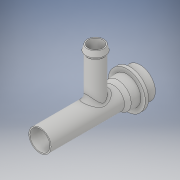
# Autodesk Inventor part: CheckBallonWindbox Connecter 1.0
Saved by Autodesk Inventor 2019 (Build 230136000, 136)
## iProperties
Created: 2019-04-04
Part Number: CheckBallonWindbox Connecter 1.0
Material: Generic
Document SubType Name: Modeling
Designer: Kepler
Density: 1 g/cm^3
Appearance: Default
Author: Kepler
Autodesk Inventor part; units mm, degrees
ref_plane "YZ Plane" through (0, 0, 0) normal (1, 0, 0) x (0, 1, 0)
ref_plane "XZ Plane" through (0, 0, 0) normal (0, 1, 0) x (-1, 0, 0)
ref_plane "XY Plane" through (0, 0, 0) normal (0, 0, 1) x (1, 0, 0)
sketch "Sketch1" plane through (0, 0, 0) normal (0, 0, 1) x (1, 0, 0)
  circle A0 centre (0, 0) radius 10
  circle A1 centre (0, 0) radius 9
  dimension "d0" = 20
  dimension "d1" = 18
  constraints: 3 coincident, 2 centre point
  measures "d0" diameter of A0
  measures "d1" diameter of A1
extrude "Extrusion1" add sketch "Sketch1" along normal blind 50
sketch "Sketch2" plane through (0, 0, 0) normal (0, 0, -1) x (-1, 0, 0)
  circle A0 centre (0, 0) radius 10
  circle A1 centre (0, 0) radius 9
  dimension "d4" = 20
  dimension "d5" = 18
  constraints: 2 centre point, 2 coincident
  measures "d4" diameter of A0
  measures "d5" diameter of A1
extrude "Extrusion2" add sketch "Sketch2" along normal blind 20
sketch "Sketch3" plane through (0, 0, 0) normal (0, 1, 0) x (-1, 0, 0)
  circle A0 centre (0, 0) radius 7.5
  circle A1 centre (0, 0) radius 6.5
  dimension "d8" = 15
  dimension "d9" = 13
  constraints: 2 centre point, 2 coincident
  measures "d8" diameter of A0
  measures "d9" diameter of A1
extrude "Extrusion3" add sketch "Sketch3" along normal blind 50
sketch "Sketch4" plane through (0, 0, 0) normal (0, -1, 0) x (1, 0, 0)
  circle A0 centre (0, 0) radius 6.5
  dimension "d12" = 13
  constraints: 1 centre point, 1 coincident
  measures "d12" diameter of A0
extrude "Extrusion4" cut sketch "Sketch4" against normal blind 20
sketch "Sketch5" plane through (0, 0, -20) normal (0, 0, -1) x (-1, 0, 0)
  circle A0 centre (0, 0) radius 9
  dimension "d15" = 18
  constraints: 1 centre point, 1 coincident
  measures "d15" diameter of A0
extrude "Extrusion5" cut sketch "Sketch5" against normal blind 30
fillet "Fillet1" radius 2 2 edges at (-0.0257, 9, 6.4999) (0.0257, 9, -6.4999)
fillet "Fillet2" radius 4 2 edges at (0.0316, 10, -7.4999) (-0.0297, 10, 7.4999)
sketch "Sketch6" plane through (0, 0, 0) normal (0, 1, 0) x (-1, 0, 0)
  line L0 (0, -20) -> (0, -40)
  line L1 (-10, -20) -> (-11.7498, -40)
  line L2 (-10, -20) -> (10, -20) projected
  line L3 (-11.7498, -40) -> (-13.7498, -40)
  line L4 (-12, -20) -> (-10, -16)
  line L5 (-10, -20) -> (-10, 50) projected
  line L6 (-10, -20) -> (-10, -16)
  line L7 (-12.6999, -28) -> (-16.6999, -28)
  line L8 (-16.6999, -28) -> (-16.6999, -31)
  line L9 (-16.6999, -31) -> (-12.9624, -31)
  line L10 (-13.7498, -40) -> (-12.9624, -31)
  line L11 (-12.6999, -28) -> (-12, -20)
  point P0 (0, 0)
  dimension "d20" = 20
  dimension "d24" = 95
  dimension "d25" = 20
  dimension "d26" = 2
  dimension "d27" = 4
  dimension "d31" = 4
  constraints: 20 end point, 2 horizontal, 2 parallel, 2 perpendicular, 1 point on line, 1 vertical
  measures "d20" distance of L0.start L0.end
  measures "d24" angle of L1 L2
  measures "d25" vertical distance of L1.start L1.end
  measures "d26" distance of L1.end L3.end
  measures "d27" vertical distance of L4.start L4.end
  measures "d31" distance of L7.start L7.end
revolve "Revolution1" add sketch "Sketch6" angle 360 about axis through (0, 0, -20) along (0, 0, -1)
sketch "Sketch7" plane through (0, 0, 0) normal (0, 0, 1) x (1, 0, 0)
  line L0 (-6.5, 50) -> (6.5, 50) projected
  line L1 (0, 50) -> (0, 44)
  line L2 (7.5, 50) -> (-7.5, 50) projected
  line L3 (7.5, 50) -> (7.5, 44)
  line L4 (7.5, 7.9844) -> (7.5, 50) projected
  line L5 (7.5, 44) -> (9, 44)
  line L6 (9, 44) -> (7.5, 50)
  point P0 (0, 0)
  constraints: 8 end point, 1 midpoint, 1 point on line, 1 vertical
revolve "Revolution2" add sketch "Sketch7" angle 360 about axis through (0, 50, 0) along (0, -1, 0)
fillet "Fillet3" radius 1 2 edges at (-9, 44, 0) (7.5, 44, 0)
body "Solid1"
